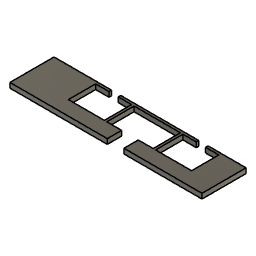
Curtains Join V2 (Autodesk Fusion 360 design; units mm, degrees)
Autodesk Fusion 360 part; units mm, degrees
sketch "Sketch1" plane through (0, 0, 0) normal (0, 0, 1) x (1, 0, 0)
  line L0 (77.5, 0) -> (77.5, 17.8)
  line L1 (0, 17.8) -> (0, 0)
  line L2 (67.5, 16.8) -> (67.5, 5.8)
  line L3 (67.5, 5.8) -> (53, 5.8)
  line L4 (53, 5.8) -> (53, 16.8)
  line L5 (32.3, 16.8) -> (32.3, 5.8)
  line L6 (32.3, 5.8) -> (17.8, 5.8)
  line L7 (17.8, 5.8) -> (17.8, 16.8)
  line L8 (25.05, 16.8) -> (25.05, 17.8) construction
  line L9 (60.25, 16.8) -> (60.25, 17.8) construction
  line L10 (58.4, 17.8) -> (58.4, 16.8)
  line L11 (62.1, 17.8) -> (62.1, 16.8)
  line L12 (23.2, 17.8) -> (23.2, 16.8)
  line L13 (26.9, 17.8) -> (26.9, 16.8)
  line L14 (52, 5.8) -> (52, 16.8)
  line L15 (52, 16.8) -> (33.3, 16.8)
  line L16 (33.3, 16.8) -> (33.3, 5.8)
  line L17 (53, 16.8) -> (58.4, 16.8)
  line L18 (62.1, 16.8) -> (67.5, 16.8)
  line L19 (77.5, 17.8) -> (62.1, 17.8)
  line L20 (17.8, 16.8) -> (23.2, 16.8)
  line L21 (26.9, 16.8) -> (32.3, 16.8)
  line L22 (58.4, 17.8) -> (26.9, 17.8)
  line L23 (23.2, 17.8) -> (0, 17.8)
  line L24 (39.3, 5.8) -> (39.3, 0)
  line L25 (46, 5.8) -> (46, 0)
  line L26 (0, 0) -> (39.3, 0)
  line L27 (46, 0) -> (77.5, 0)
  line L28 (33.3, 5.8) -> (39.3, 5.8)
  line L29 (46, 5.8) -> (52, 5.8)
  dimension "d1" = 77.5
  dimension "d2" = 17.8
  dimension "d9" = 14.5
  dimension "d10" = 11
  dimension "d11" = 10
  dimension "d12" = 1
  dimension "d13" = 14.5
  dimension "d14" = 11
  dimension "d15" = 17.8
  dimension "d16" = 1
  dimension "d18" = 20.7
  dimension "d19" = 1.85
  dimension "d20" = 1.85
  dimension "d21" = 1.85
  dimension "d22" = 1.85
  dimension "d23" = 1
  dimension "d24" = 1
  dimension "d25" = 11
  dimension "d26" = 1
  dimension "d27" = 6
  dimension "d28" = 6
  constraint horizontal L26
  constraint vertical L0
  constraint horizontal L19
  constraint vertical L1
  constraint coincident L1.end L26.start
  constraint horizontal L17
  constraint vertical L2
  constraint horizontal L3
  constraint vertical L4
  constraint horizontal L20
  constraint vertical L5
  constraint horizontal L6
  constraint vertical L7
  constraint coincident L8.end L19
  constraint perpendicular L8 L19
  constraint coincident L9.end L19
  constraint perpendicular L9 L19
  constraint coincident L10.start L19
  constraint perpendicular L10 L17
  constraint coincident L11.end L17
  constraint perpendicular L11 L17
  constraint coincident L12.start L19
  constraint perpendicular L12 L20
  constraint coincident L13.start L19
  constraint coincident L13.end L20
  constraint perpendicular L13 L20
  constraint horizontal L28
  constraint vertical L14
  constraint horizontal L15
  constraint vertical L16
  constraint collinear L17 L18
  constraint coincident L9.start L17
  constraint collinear L19 L22
  constraint collinear L20 L21
  constraint coincident L8.start L20
  constraint collinear L22 L23
  constraint perpendicular L24 L26
  constraint coincident L25.start L28
  constraint coincident L25.end L26
  constraint perpendicular L25 L26
  constraint collinear L26 L27
  constraint collinear L28 L29
  measures "d1" distance of L1.end L0.start
  measures "d2" distance of L1.end L1.start
  measures "d9" distance of L4.end L2.start
  measures "d10" distance of L4.end L3.end
  measures "d11" distance of L0 L2
  measures "d12" distance of L17 L19
  measures "d13" distance of L7.end L5.start
  measures "d14" distance of L7.end L6.end
  measures "d15" distance of L1 L7
  measures "d16" distance of L19 L20
  measures "d18" distance of L4 L5
  measures "d19" distance of L9 L11
  measures "d20" distance of L9 L10
  measures "d21" distance of L8 L13
  measures "d22" distance of L8 L12
  measures "d23" distance of L5 L16
  measures "d24" distance of L4 L14
  measures "d25" distance of L15 L28
  measures "d26" distance of L15 L19
  measures "d27" distance of L16.end L24
  measures "d28" distance of L14.start L25
extrude "Extrude1" add sketch "Sketch1" along normal blind 2
equation "d19 = ( 3.7 / 2 ) * 1 mm"
equation "d20 = ( 3.7 / 2 ) * 1 mm"
equation "d21 = ( 3.7 / 2 ) * 1 mm"
equation "d22 = ( 3.7 / 2 ) * 1 mm"
